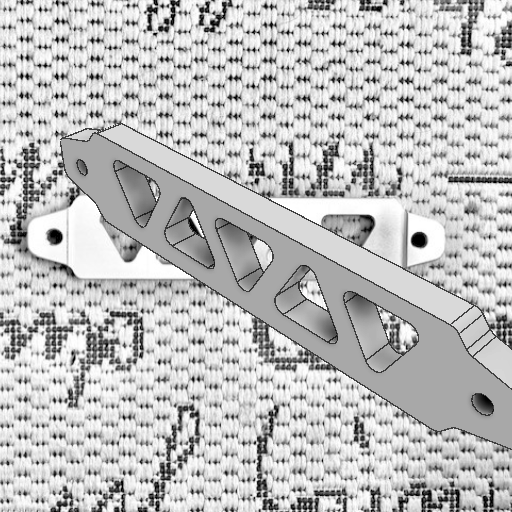
# Autodesk Inventor part: BatteryMount
Saved by Autodesk Inventor 2025.2 (Build 292293000, 293)
## iProperties
Created: 2026-05-27
Part Number: BatteryMount
Material: Generic
Document SubType Name: Modeling
Designer: valer
Density: 1 g/cm^3
Appearance: Default
Author: valer
Autodesk Inventor part; units mm, degrees
ref_plane "YZ Plane" through (0, 0, 0) normal (1, 0, 0) x (0, 1, 0)
ref_plane "XZ Plane" through (0, 0, 0) normal (0, 1, 0) x (-1, 0, 0)
ref_plane "XY Plane" through (0, 0, 0) normal (0, 0, 1) x (1, 0, 0)
sketch "Base" plane through (0, 0, 0) normal (0, 0, 1) x (1, 0, 0)
  line L0 (-152.6, 0) -> (152.6, 0) construction
  line L1 (0, -28.7) -> (0, 28.7) construction
  circle A0 centre (-95, 0) radius 3.5
  circle A1 centre (95, 0) radius 3.5
  line L2 (-109, 8.7447) -> (-109, 0)
  line L3 (-109, 8.7447) -> (-88, 14.3716)
  line L4 (-88, 14.3716) -> (-82.8577, 20.5)
  line L5 (-82.8577, 20.5) -> (0, 20.5)
  line L6 (-109, -8.7447) -> (-109, 0)
  line L7 (-109, -8.7447) -> (-88, -14.3716)
  line L8 (-88, -14.3716) -> (-82.8577, -20.5)
  line L9 (-82.8577, -20.5) -> (0, -20.5)
  line L10 (109, 8.7447) -> (109, 0)
  line L11 (109, 8.7447) -> (88, 14.3716)
  line L12 (88, 14.3716) -> (82.8577, 20.5)
  line L13 (82.8577, 20.5) -> (0, 20.5)
  line L14 (82.8577, -20.5) -> (0, -20.5)
  line L15 (88, -14.3716) -> (82.8577, -20.5)
  line L16 (109, -8.7447) -> (88, -14.3716)
  line L17 (109, -8.7447) -> (109, 0)
  circle A2 centre (-68, 9.5) radius 4
  line L18 (-58, 0) -> (-58, 20.5) construction
  line L19 (-68, 13.5) -> (-58, 13.5)
  circle A3 centre (-58, -7.8205) radius 4
  line L20 (-58, 0) -> (-58, -7.8205) construction
  line L21 (-71.4641, 7.5) -> (-61.4641, -9.8205)
  circle A4 centre (-48, 9.5) radius 4
  line L22 (-58, 13.5) -> (-48, 13.5)
  line L23 (-54.5359, -9.8205) -> (-44.5359, 7.5)
  circle A5 centre (-29, 9.5) radius 4
  circle A6 centre (-39, -7.8205) radius 4
  circle A7 centre (-19, -7.8205) radius 4
  line L24 (-48, 13.5) -> (-29, 13.5) construction
  line L25 (-39, -11.8205) -> (-19, -11.8205)
  line L26 (-42.4641, -5.8205) -> (-32.4641, 11.5)
  line L27 (-25.5359, 11.5) -> (-15.5359, -5.8205)
  line L28 (-58, -11.8205) -> (-39, -11.8205) construction
  line L29 (-29, 9.5) -> (-29, -11.8205) construction
  circle A8 centre (10, 9.5) radius 4
  line L30 (10, 13.5) -> (0, 13.5)
  circle A9 centre (0, -7.8205) radius 4
  line L31 (13.4641, 7.5) -> (3.4641, -9.8205)
  circle A10 centre (-10, 9.5) radius 4
  line L32 (0, 13.5) -> (-10, 13.5)
  line L33 (-3.4641, -9.8205) -> (-13.4641, 7.5)
  circle A11 centre (68, 9.5) radius 4
  line L34 (68, 13.5) -> (58, 13.5)
  circle A12 centre (58, -7.8205) radius 4
  line L35 (71.4641, 7.5) -> (61.4641, -9.8205)
  circle A13 centre (48, 9.5) radius 4
  line L36 (58, 13.5) -> (48, 13.5)
  line L37 (54.5359, -9.8205) -> (44.5359, 7.5)
  circle A14 centre (29, 9.5) radius 4
  circle A15 centre (39, -7.8205) radius 4
  circle A16 centre (19, -7.8205) radius 4
  line L38 (39, -11.8205) -> (19, -11.8205)
  line L39 (42.4641, -5.8205) -> (32.4641, 11.5)
  line L40 (25.5359, 11.5) -> (15.5359, -5.8205)
  point P0 (0, 0)
  point P1 (-58, 10.25)
  dimension "d0" = 7
  dimension "d1" = 190
  dimension "d3" = 130
  dimension "d4" = 165
  dimension "d5" = 8
  dimension "d7" = 218
  dimension "d8" = 41
  dimension "d12" = 21
  dimension "d14" = 8
  dimension "d15" = 8
  dimension "d16" = 20
  dimension "d17" = 60
  dimension "d18" = 7
  dimension "d20" = 8.4545
  dimension "d21" = 8.4545
  constraints: 78 end point, 42 symmetric about line, 32 point on circle, 17 centre point, 15 tangent, 8 point on line, 3 equal radius, 3 perpendicular, 2 midpoint, 2 parallel, 2 vertical, 1 collinear, 1 horizontal, 11 other
  measures "d0" diameter of A0
  measures "d1" distance of A1.centre A0.centre
  measures "d3" angle of L5 L4
  measures "d4" angle of L5 L3
  measures "d5" distance of L3.end L4.end
  measures "d7" distance between parallel lines of L10 L2
  measures "d8" distance between parallel lines of L9 L5
  measures "d12" horizontal distance of L2.start L3.end
  measures "d14" diameter of A2
  measures "d15" diameter of A3
  measures "d16" distance of A4.centre A2.centre
  measures "d17" angle of L21 L19
  measures "d18" distance between parallel lines of L5 L19
  measures "d20" distance between parallel lines of L26 L23
  measures "d21" distance between parallel lines of L33 L27
extrude "BaseFeature" add sketch "Base" along normal blind 12
fillet "OutsideFilletsFeature" radius 4 12 edges at (-109, -8.7447, 6) (-109, 8.7447, 6) (-88, -14.3716, 6) (-82.8577, -20.5, 6) (-88, 14.3716, 6) (-82.8577, 20.5, 6) (82.8577, 20.5, 6) (88, 14.3716, 6) (109, -8.7447, 6) (88, -14.3716, 6) (82.8577, -20.5, 6) (109, 8.7447, 6)
body "Solid1"
